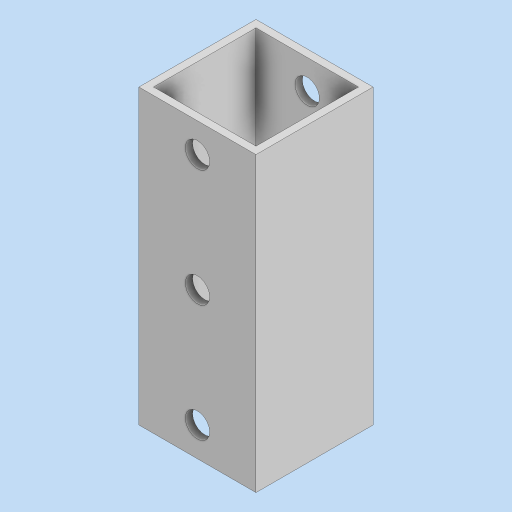
# Autodesk Inventor part: 2.5inTube
Saved by Autodesk Inventor 2024 (Build 280153000, 153)
## iProperties
Created: 2023-11-16
Part Number: 2.5inTube
Material: Generic
Document SubType Name: Modeling
Designer: megan
Density: 1 g/cm^3
Appearance: Default
Author: megan
Autodesk Inventor part; units mm, degrees
ref_plane "YZ Plane" through (0, 0, 0) normal (1, 0, 0) x (0, 1, 0)
ref_plane "XZ Plane" through (0, 0, 0) normal (0, 1, 0) x (-1, 0, 0)
ref_plane "XY Plane" through (0, 0, 0) normal (0, 0, 1) x (1, 0, 0)
sketch "Sketch1" plane through (0, 0, 0) normal (0, 1, 0) x (-1, 0, 0)
  line L0 (0, 0) -> (25.4, 0)
  line L1 (25.4, 0) -> (25.4, -25.4)
  line L2 (25.4, -25.4) -> (0, -25.4)
  line L3 (0, -25.4) -> (0, 0)
  line L4 (23.8125, -1.5875) -> (1.5875, -1.5875)
  line L5 (1.5875, -1.5875) -> (1.5875, -23.8125)
  line L6 (1.5875, -23.8125) -> (23.8125, -23.8125)
  line L7 (23.8125, -23.8125) -> (23.8125, -1.5875)
  dimension "d0" = 25.4
  dimension "d1" = 25.4
  dimension "d2" = 1.5875
  dimension "d3" = 1.5875
  dimension "d4" = 1.5875
  dimension "d5" = 1.5875
  constraints: 16 end point, 4 parallel, 2 horizontal, 2 perpendicular
  measures "d0" distance of L1.end L2.end
  measures "d1" distance of L0.end L1.end
  measures "d2" distance between parallel lines of L1 L7
  measures "d3" distance between parallel lines of L0 L4
  measures "d4" distance between parallel lines of L3 L5
  measures "d5" distance between parallel lines of L2 L6
extrude "Extrusion1" add sketch "Sketch1" along normal blind 63.5
sketch "Sketch2" plane through (-25.4, 0, 0) normal (0, 0, 1) x (1, 0, 0)
  line L0 (1.5875, 63.5) -> (23.8125, 63.5) construction
  line L1 (12.7, 63.5) -> (12.7, 0) construction
  line L2 (23.8125, 0) -> (1.5875, 0) construction
  line L3 (0, 0) -> (0, 63.5) construction
  line L4 (0, 31.75) -> (25.4, 31.75) construction
  circle A0 centre (12.7, 31.75) radius 2.65
  circle A1 centre (12.7, 57.15) radius 2.65
  circle A2 centre (12.7, 6.35) radius 2.65
  point P0 (25.4, 0)
  point P1 (12.7, 31.75)
  dimension "d8" = 5.3
  dimension "d9" = 25.4
  dimension "d10" = 25.4
  constraints: 5 midpoint, 4 end point, 3 centre point, 2 equal radius, 2 point on line, 1 horizontal
  measures "d8" diameter of A0
  measures "d9" distance of A1.centre point (12.7, 31.75)
  measures "d10" distance of A0.centre A2.centre
extrude "Extrusion2" cut sketch "Sketch2" against normal through all
body "Solid1"
